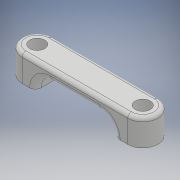
# Autodesk Inventor part: cable clip
Saved by Autodesk Inventor 2017 (Build 210142000, 142)
## iProperties
Created: 2018-09-04
Part Number: cable clip
Material: Generic
Document SubType Name: Modeling
Designer: jakub.tomczynski
Density: 1 g/cm^3
Appearance: Default
Author: jakub.tomczynski
## iProperties of the stored document cable clip_3DPrint.ipt
Created: 2018-09-05
Part Number: cable clip_3DPrint
Material: Generic
Document SubType Name: Modeling
Designer: jakub.tomczynski
Density: 1 g/cm^3
Appearance: Default
Author: jakub.tomczynski
Autodesk Inventor part; units mm, degrees
ref_plane "YZ Plane" through (0, 0, 0) normal (1, 0, 0) x (0, 1, 0)
ref_plane "XZ Plane" through (0, 0, 0) normal (0, 1, 0) x (-1, 0, 0)
ref_plane "XY Plane" through (0, 0, 0) normal (0, 0, 1) x (1, 0, 0)
sketch "Sketch1" plane through (0, 0, 0) normal (0, 0, 1) x (1, 0, 0)
  line L0 (-14, 0) -> (14, 0) construction
  line L1 (-14, -4) -> (14, -4)
  line L2 (14, 4) -> (-14, 4)
  arc A0 (-14, 4) -> (-14, -4) centre (-14, 0) ccw
  arc A1 (14, -4) -> (14, 4) centre (14, 0) ccw
  point P0 (0, 0)
  dimension "d0" = 8
  dimension "d1" = 28
  constraints: 8 end point, 4 point on circle, 4 tangent, 2 centre point, 1 horizontal, 1 midpoint, 1 parallel
  measures "d0" distance between parallel lines of L1 L2
  measures "d1" distance of L0.end L0.start
extrude "Extrusion1" add sketch "Sketch1" along normal blind 7
sketch "Sketch2" plane through (-14, -4, 0) normal (0, -1, 0) x (1, 0, 0)
  line L0 (7.5, 0) -> (20.5, 0) construction
  line L1 (7.5, -4) -> (20.5, -4)
  line L2 (20.5, 4) -> (7.5, 4)
  arc A0 (7.5, 4) -> (7.5, -4) centre (7.5, 0) ccw
  arc A1 (20.5, -4) -> (20.5, 4) centre (20.5, 0) ccw
  point P0 (14, 0)
  dimension "d4" = 4
  dimension "d5" = 13
  constraints: 8 end point, 4 point on circle, 4 tangent, 2 centre point, 1 horizontal, 1 midpoint, 1 parallel
  measures "d4" distance between parallel lines of L2 L0
  measures "d5" distance of L0.end L0.start
extrude "Extrusion2" cut sketch "Sketch2" against normal through all
fillet "Fillet1" radius 1.5 6 edges at (0, -4, 4) (9.3284, -4, 2.8284) (-9.3284, -4, 2.8284) (0, 4, 4) (9.3284, 4, 2.8284) (-9.3284, 4, 2.8284)
fillet "Fillet2" radius 1 4 edges at (18, 0, 7) (0, 4, 7) (-18, 0, 7) (0, -4, 7)
sketch "Sketch3" plane through (0, 0, 7) normal (0, 0, 1) x (1, 0, 0)
  arc A0 (14, -4) -> (14, 4) centre (14, 0) ccw projected
  arc A1 (-14, 4) -> (-14, -4) centre (-14, 0) ccw projected
  point P0 (0, 0)
hole "Hole1" at (14, 0, 7) at (-14, 0, 7) direction (0, 0, -1) diameter 1.9 end through all counterbore diameter 4 counterbore depth 4
body "Solid1"
